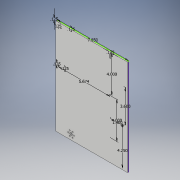
# Autodesk Inventor part: ElectronicsPlate
Saved by Autodesk Inventor 2017 (Build 210142000, 142)
## iProperties
Created: 2018-01-06
Part Number: ElectronicsPlate
Material: Generic
Document SubType Name: Modeling
Designer: User
Density: 1 g/cm^3
Appearance: Default
Author: User
Autodesk Inventor part; units mm, degrees
ref_plane "YZ Plane" through (0, 0, 0) normal (1, 0, 0) x (0, 1, 0)
ref_plane "XZ Plane" through (0, 0, 0) normal (0, 1, 0) x (-1, 0, 0)
ref_plane "XY Plane" through (0, 0, 0) normal (0, 0, 1) x (1, 0, 0)
sketch "Sketch1" plane through (0, 0, 0) normal (0, 0, 1) x (1, 0, 0)
  line L0 (0, 0) -> (199.39, 0)
  line L1 (199.39, 0) -> (199.39, 266.7)
  line L2 (199.39, 266.7) -> (0, 266.7)
  line L3 (0, 266.7) -> (0, 0)
  line L4 (12.1493, 266.7) -> (12.1493, 263.525)
  line L5 (0, 247.1772) -> (3.175, 247.1772)
  line L6 (3.175, 263.525) -> (147.2946, 263.525)
  line L7 (147.2946, 263.525) -> (147.2946, 161.925)
  line L8 (147.2946, 161.925) -> (3.175, 161.925)
  line L9 (3.175, 161.925) -> (3.175, 263.525)
  line L10 (5.8968, 161.925) -> (5.8968, 158.75)
  line L11 (3.175, 158.75) -> (147.2946, 158.75)
  line L12 (147.2946, 158.75) -> (147.2946, 57.15)
  line L13 (147.2946, 57.15) -> (3.175, 57.15)
  line L14 (3.175, 57.15) -> (3.175, 158.75)
  line L15 (147.2946, 247.6224) -> (150.4696, 247.6224)
  line L16 (150.4696, 199.39) -> (186.0296, 199.39)
  line L17 (186.0296, 199.39) -> (186.0296, 107.95)
  line L18 (186.0296, 107.95) -> (150.4696, 107.95)
  line L19 (150.4696, 107.95) -> (150.4696, 199.39)
  dimension "d0" = 199.39
  dimension "d2" = 3.175
  dimension "d3" = 3.175
  dimension "d4" = 144.1196
  dimension "d5" = 101.6
  dimension "d6" = 3.175
  dimension "d7" = 101.6
  dimension "d8" = 3.175
  dimension "d9" = 35.56
  dimension "d10" = 91.44
  dimension "d11" = 107.95
  dimension "d12" = 3.175
  dimension "d13" = 3.175
  constraints: 40 end point, 8 parallel, 7 perpendicular, 5 horizontal, 4 point on line
  measures "d0" distance of L2.end L1.end
  measures "d2" distance of L4.start L4.end
  measures "d3" distance of L5.start L5.end
  measures "d4" distance of L7.end L8.end
  measures "d5" distance of L6.end L7.end
  measures "d6" distance of L10.start L10.end
  measures "d7" distance of L11.end L12.end
  measures "d8" distance of L15.start L15.end
  measures "d9" distance of L17.end L18.end
  measures "d10" distance of L16.end L17.end
  measures "d11" distance between parallel lines of L0 L18
  measures "d12" distance between parallel lines of L2 L6
  measures "d13" distance between parallel lines of L8 L11
sketch "Sketch2" plane through (0, 0, 0) normal (0, 0, 1) x (1, 0, 0)
  line L0 (199.39, 0) -> (0, 0)
  line L1 (0, 0) -> (0, 266.7)
  line L2 (0, 266.7) -> (199.39, 266.7)
  line L3 (199.39, 266.7) -> (199.39, 0)
  point P0 (0, 0)
  constraints: 8 end point, 2 parallel, 1 horizontal, 1 perpendicular
extrude "Extrusion1" add sketch "Sketch2" along normal blind 3.175
sketch "Sketch3" plane through (0, 0, 3.175) normal (0, 0, 1) x (1, 0, 0)
  line L0 (33.6942, 0) -> (33.6942, 14.605)
  line L1 (0, 14.605) -> (42.5196, 14.605)
  line L2 (0, 14.605) -> (42.5196, 14.605) construction
  circle A0 centre (42.5196, 14.605) radius 8.001
  circle A1 centre (42.5196, 14.605) radius 3.4925
  circle A2 centre (34.5186, 14.605) radius 1.5875
  circle A3 centre (38.5191, 7.6759) radius 1.5875
  circle A4 centre (46.5201, 7.6759) radius 1.5875
  circle A5 centre (50.5206, 14.605) radius 1.5875
  circle A6 centre (46.5201, 21.5341) radius 1.5875
  circle A7 centre (38.5191, 21.5341) radius 1.5875
  dimension "d20" = 16.002
  dimension "d16" = 14.605
  dimension "d18" = 42.5196
  dimension "d19" = 0
  dimension "d21" = 6.985
  dimension "d22" = 3.175
  dimension "d27" = 360
  constraints: 7 centre point, 6 end point, 2 coincident, 1 collinear, 1 horizontal, 1 horizontal alignment, 1 point on line, 15 other
  measures "d16" distance of L0.start L0.end
  measures "d18" distance of L1.start L1.end
  measures "d19" distance between parallel lines of L1 L2
  measures "d21" diameter of A1
  measures "d22" diameter of A2
extrude "Extrusion2" cut sketch "Sketch3" against normal blind 6.35 contours A2 L1 L0 | L0 L1 A0 A2 | L1 A2 A0 | A0 L1 A2 | A0 A2 L1 | A3 A0 | A0 A3 | A7 A0 | A0 A7 | A4 A0 | A0 A4 | A6 A0 | A0 A6 | A5 A0 | A0 A5 | A1
body "Solid1"
